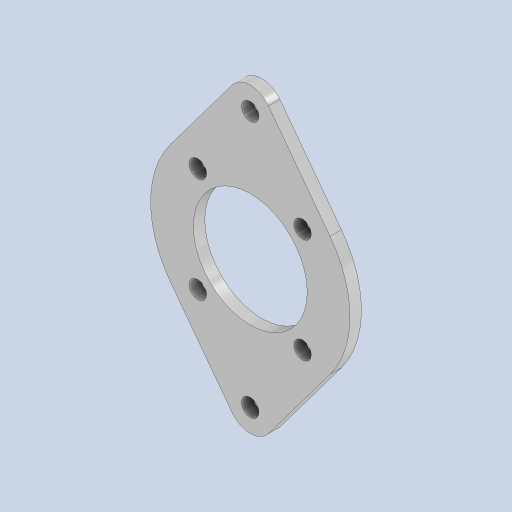
# Autodesk Inventor part: al_motorbase_1
Saved by Autodesk Inventor 2024 (Build 280153000, 153)
## iProperties
Created: 2023-03-18
Part Number: al_motorbase_1
Material: アルミニウム 6061-AHC
Document SubType Name: Modeling
Designer: blueh
Density: 2.7 g/cm^3
Appearance: アルミニウム - ダーク
Author: blueh
Autodesk Inventor part; units mm, degrees
ref_plane "YZ Plane" through (0, 0, 0) normal (1, 0, 0) x (0, 1, 0)
ref_plane "XZ Plane" through (0, 0, 0) normal (0, 1, 0) x (-1, 0, 0)
ref_plane "XY Plane" through (0, 0, 0) normal (0, 0, 1) x (1, 0, 0)
sketch "スケッチ1" plane through (0, 0, 0) normal (0, 0, 1) x (1, 0, 0)
  circle A0 centre (0, 0) radius 10
  circle A1 centre (0, 0) radius 13 construction
  line L0 (0, 0) -> (0, -7.3396) construction
  circle A2 centre (9.1924, -9.1924) radius 1.55 construction
  line L1 (0, 0) -> (9.1924, -9.1924) construction
  circle A3 centre (9.1924, 9.1924) radius 1.55 construction
  circle A4 centre (-9.1924, 9.1924) radius 1.55 construction
  circle A5 centre (-9.1924, -9.1924) radius 1.55 construction
  line L2 (-24.5, 0) -> (24.5, 0) projected
  circle A6 centre (0, 22.5) radius 4
  circle A7 centre (0, -22.5) radius 4
  circle A8 centre (0, 0) radius 16 construction
  circle A9 centre (0, 0) radius 17.5
  line L3 (-3.2, 24.9) -> (-14, 10.5)
  line L4 (-3.2, -24.9) -> (-14, -10.5)
  line L5 (3.2, -24.9) -> (14, -10.5)
  line L6 (3.2, 24.9) -> (14, 10.5)
  dimension "d3" = 26
  dimension "d2" = 20
  dimension "d4" = 3.1
  dimension "d5" = 45
  dimension "d9" = 360
  dimension "d13" = 45
  dimension "d14" = 8
  dimension "d15" = 8
  dimension "d16" = 32
  dimension "d17" = 35
  constraints: 12 end point, 11 coincident, 9 centre point, 8 point on circle, 8 tangent, 1 symmetric about line, 1 vertical, 1 vertical alignment, 16 other
  measures "d2" diameter of A0
  measures "d4" diameter of A2
  measures "d5" angle of L1 L0
  measures "d13" distance of point (0, -22.5) point (0, 22.5)
  measures "d14" diameter of A6
  measures "d15" diameter of A7
  measures "d16" diameter of A8
  measures "d17" diameter of A9
extrude "押し出し1" add sketch "スケッチ1" along normal blind 2 contours L2 A9 A0 | A0 L2 A9 | A9 L3 A6 L6 | L5 A7 L4 A9 | A6 | A7
hole "穴1" at (9.1924, -9.1924, 0) at (-9.1924, -9.1924, 0) at (9.1924, 9.1924, 0) at (-9.1924, 9.1924, 0) at (0, 22.5, 0) at (0, -22.5, 0) direction (0, 0, 1) diameter 3.05 end through all
